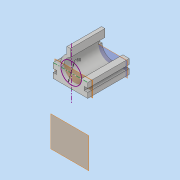
# Autodesk Inventor part: lw_3_ползунок
Saved by Autodesk Inventor 2019 (Build 230136000, 136)
## iProperties
Created: 2021-02-21
Part Number: lw_3_ползунок
Material: Типовые
Document SubType Name: Modeling
Designer: Kurbatova
Density: 1 g/cm^3
Appearance: По умолчанию
Author: Kurbatova
Autodesk Inventor part; units mm, degrees
ref_plane "YZ Plane" through (0, 0, 0) normal (1, 0, 0) x (0, 1, 0)
ref_plane "XZ Plane" through (0, 0, 0) normal (0, 1, 0) x (-1, 0, 0)
ref_plane "XY Plane" through (0, 0, 0) normal (0, 0, 1) x (1, 0, 0)
sketch "Эскиз1" plane through (0, 0, 0) normal (0, 1, 0) x (-1, 0, 0)
  line L0 (53.8137, 54.0949) -> (-46.1863, 54.0949)
  line L1 (-46.1863, 54.0949) -> (-46.1863, -65.9051)
  line L2 (-46.1863, -65.9051) -> (53.8137, -65.9051)
  line L3 (53.8137, -65.9051) -> (53.8137, 54.0949)
  line L4 (102.7933, -5.9051) -> (-137.2052, -5.9051)
  point P0 (0, 0)
  point P1 (53.8137, -5.9051)
  dimension "d0" = 120
  dimension "d1" = 100
  constraints: 10 end point, 2 horizontal, 2 parallel, 1 midpoint, 1 perpendicular, 1 point on line
  measures "d0" distance between parallel lines of L2 L0
  measures "d1" distance between parallel lines of L1 L3
extrude "Выдавливание1" add sketch "Эскиз1" along normal blind 40
sketch "Эскиз2" plane through (-53.8137, 0, 54.0949) normal (0, 0, 1) x (1, 0, 0)
  circle A0 centre (51.5912, 40) radius 30
  line L0 (51.5912, 113.4013) -> (51.5912, -34.7388)
  line L1 (0, 40) -> (100, 40) projected
  point P0 (53.8137, 0)
  dimension "d6" = 60
  constraints: 2 end point, 2 point on line, 1 centre point, 1 vertical
  measures "d6" diameter of A0
extrude "Углубление 1" cut sketch "Эскиз2" against normal blind 120
sketch "Эскиз4" plane through (-53.8137, 0, 54.0949) normal (0, 0, 1) x (1, 0, 0)
  line L0 (0, 0) -> (100, 0) projected
  line L1 (-0.0635, 15) -> (9.9365, 15)
  line L2 (9.9365, 15) -> (9.9365, 25)
  line L3 (9.9365, 25) -> (-0.0635, 25)
  line L4 (-0.0635, 25) -> (-0.0635, 15)
  line L5 (0, 40) -> (21.5912, 40) projected
  line L6 (89.6996, 15) -> (99.6996, 15)
  line L7 (99.6996, 15) -> (99.6996, 25)
  line L8 (99.6996, 25) -> (89.6996, 25)
  line L9 (89.6996, 25) -> (89.6996, 15)
  point P0 (53.8137, 0)
  dimension "d11" = 10
  dimension "d12" = 10
  dimension "d13" = 15
  dimension "d14" = 15
  dimension "d15" = 40
  dimension "d16" = 10
  dimension "d17" = 10
  dimension "d18" = 15
  constraints: 18 end point, 6 perpendicular, 2 horizontal
  measures "d11" distance between parallel lines of L1 L3
  measures "d12" distance between parallel lines of L2 L4
  measures "d13" distance between parallel lines of L0 L1
  measures "d14" distance between parallel lines of L3 L5
  measures "d15" distance between parallel lines of L0 L5
  measures "d16" distance between parallel lines of L6 L8
  measures "d17" distance between parallel lines of L7 L9
  measures "d18" distance between parallel lines of L0 L6
extrude "Паз 1" cut sketch "Эскиз4" against normal up to next contours L4 L3 L2 L1
sketch "Эскиз6" plane through (-53.8137, 0, 54.0949) normal (0, 0, 1) x (1, 0, 0)
  line L0 (0, 0) -> (100, 0)
  line L1 (-0.0635, 15) -> (9.9365, 15)
  line L2 (9.9365, 15) -> (9.9365, 25)
  line L3 (9.9365, 25) -> (-0.0635, 25)
  line L4 (-0.0635, 25) -> (-0.0635, 15)
  line L5 (0, 40) -> (12.829, 40)
  line L6 (100, 25) -> (90, 25)
  line L7 (100, 15) -> (100, 25)
  line L8 (90, 25) -> (90, 15)
  line L9 (90, 15) -> (100, 15)
  line L10 (100, 0) -> (100, 40) projected
  point P0 (53.8137, 0)
  point P1 (53.8137, 0)
  dimension "d21" = 10
  dimension "d22" = 10
  dimension "d23" = 15
  dimension "d24" = 15
  dimension "d25" = 40
  dimension "d26" = 10
  dimension "d27" = 10
  dimension "d28" = 15
  constraints: 22 end point, 6 perpendicular, 2 horizontal, 1 collinear
  measures "d21" distance between parallel lines of L1 L3
  measures "d22" distance between parallel lines of L2 L4
  measures "d23" distance between parallel lines of L0 L1
  measures "d24" distance between parallel lines of L3 L5
  measures "d25" distance between parallel lines of L0 L5
  measures "d26" distance between parallel lines of L9 L6
  measures "d27" distance between parallel lines of L7 L8
  measures "d28" distance between parallel lines of L0 L9
extrude "Паз 2" cut sketch "Эскиз6" against normal up to next contours L7 L9 L8 L6
ref_plane "фронт1" through (-53.8137, 0, 44.0949) normal (0, 0, 1) x (1, 0, 0)
ref_plane "фронт2" through (46.1863, 0, -55.9051) normal (0, 0, -1) x (-1, 0, 0)
sketch "Эскиз10" plane through (-53.8137, 0, 44.0949) normal (0, 0, 1) x (1, 0, 0)
  line L0 (39.8085, 90) -> (29.8085, 90)
  line L1 (29.8085, 90) -> (29.8085, 71.2836)
  line L2 (59.8085, 90) -> (59.8085, 68.7728)
  line L3 (59.8085, 90) -> (69.8085, 90)
  line L4 (69.8085, 90) -> (69.8085, 73.2683)
  arc A0 (21.5912, 40) -> (81.5912, 40) centre (51.5912, 40) ccw projected
  arc A1 (39.8085, 67.5893) -> (21.5912, 40) centre (51.5912, 40) ccw
  line L5 (39.8085, 67.5893) -> (39.8085, 90)
  arc A2 (81.5703, 39.7664) -> (59.8085, 68.7728) centre (51.6179, 39.9614) ccw
  line L6 (21.5912, 40) -> (11.5912, 40)
  arc A3 (29.8085, 71.2836) -> (11.5912, 40) centre (51.5245, 37.6917) ccw
  line L7 (81.5912, 40) -> (91.5912, 40)
  arc A4 (91.5912, 40) -> (69.8085, 73.2683) centre (51.3632, 37.4258) ccw
  point P0 (53.8137, 0)
  dimension "d59" = 20
  dimension "d60" = 10
  dimension "d61" = 10
  dimension "d63" = 10
  dimension "d64" = 40
  dimension "d70" = 10
  dimension "d71" = 50
  dimension "d72" = 50
  constraints: 16 end point, 8 point on circle, 4 centre point, 3 horizontal, 2 perpendicular, 2 tangent, 2 vertical
  measures "d59" distance between parallel lines of L2 L5
  measures "d60" distance between parallel lines of L5 L1
  measures "d61" distance between parallel lines of L2 L4
  measures "d63" distance of L6.start L6.end
  measures "d64" radius of A3
  measures "d70" distance of L7.start L7.end
  measures "d71" distance from line of L6.end L0
  measures "d72" distance between parallel lines of L7 L3
extrude "Выдавливание5" add sketch "Эскиз10" against normal up to surface (100 mm away)
sketch "Эскиз13" plane through (-53.8137, 0, 44.0949) normal (0, 0, 1) x (1, 0, 0)
  point P0 (53.8137, 0)
sketch "Эскиз14" plane through (-53.8137, 0, 44.0949) normal (0, 0, 1) x (1, 0, 0)
  point P0 (53.8137, 0)
ref_plane "РабПлоскость16" through (-53.8137, 0, 49.0949) normal (0, 0, 1) x (1, 0, 0)
